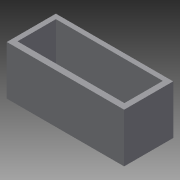
# Autodesk Inventor part: Fader Cap
Saved by Autodesk Inventor 2015 (Build 190159000, 159)
## iProperties
Created: 2016-04-25
Part Number: Fader Cap
Material: Generic
Document SubType Name: Modeling
Designer: HP USER
Density: 1 g/cm^3
Appearance: Default
Author: HP USER
Autodesk Inventor part; units mm, degrees
ref_plane "YZ Plane" through (0, 0, 0) normal (1, 0, 0) x (0, 1, 0)
ref_plane "XZ Plane" through (0, 0, 0) normal (0, 1, 0) x (-1, 0, 0)
ref_plane "XY Plane" through (0, 0, 0) normal (0, 0, 1) x (1, 0, 0)
sketch "Sketch1" plane through (0, 0, 0) normal (0, 0, 1) x (1, 0, 0)
  line L0 (0, 0) -> (22, 0)
  line L1 (22, 0) -> (22, -9.2)
  line L2 (22, -9.2) -> (0, -9.2)
  line L3 (0, -9.2) -> (0, 0)
  dimension "d0" = 22
  dimension "d1" = 9.2
  constraints: 8 end point
  measures "d0" distance of L1.end L2.end
  measures "d1" distance of L0.end L1.end
extrude "Extrusion1" add sketch "Sketch1" along normal blind 9.2
sketch "Sketch2" plane through (0, 0, 9.2) normal (0, 0, 1) x (1, 0, 0)
  line L0 (0.9024, -0.8915) -> (20.9524, -0.8915)
  line L1 (20.9524, -0.8915) -> (20.9524, -8.0915)
  line L2 (20.9524, -8.0915) -> (0.9024, -8.0915)
  line L3 (0.9024, -8.0915) -> (0.9024, -0.8915)
  point P0 (0, 0)
  dimension "d4" = 20.05
  dimension "d5" = 7.2
  constraints: 8 end point
  measures "d4" distance of L1.end L2.end
  measures "d5" distance of L0.end L1.end
extrude "Extrusion2" cut sketch "Sketch2" against normal blind 7.2
sketch "Sketch3" plane through (0, 0, 0) normal (0, 0, -1) x (-1, 0, 0)
  circle A0 centre (-10.8985, -4.6543) radius 1.435
  point P0 (0, 0)
  dimension "d8" = 2.87
  constraints: 1 centre point
  measures "d8" diameter of A0
extrude "Extrusion3" cut sketch "Sketch3" against normal blind 7.2
body "Solid1"
